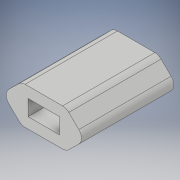
# Autodesk Inventor part: USB Plug Protector
Saved by Autodesk Inventor 2019 (Build 230136000, 136)
## iProperties
Created: 2021-08-13
Part Number: USB Plug Protector
Material: Generic
Document SubType Name: Modeling
Designer: Lix
Density: 1 g/cm^3
Appearance: Default
Author: Lix
Autodesk Inventor part; units mm, degrees
ref_plane "YZ Plane" through (0, 0, 0) normal (1, 0, 0) x (0, 1, 0)
ref_plane "XZ Plane" through (0, 0, 0) normal (0, 1, 0) x (-1, 0, 0)
ref_plane "XY Plane" through (0, 0, 0) normal (0, 0, 1) x (1, 0, 0)
sketch "Sketch1" plane through (0, 0, 0) normal (0, 0, 1) x (1, 0, 0)
  line L0 (-9.5418, 7) -> (9.5418, 7) construction
  arc A0 (-9.5418, 7) -> (-10.9418, 6.4283) centre (-9.5418, 5) ccw construction
  line L1 (-16.0429, 1.4283) -> (-10.9418, 6.4283) construction
  arc A1 (-16.0429, 1.4283) -> (-16.0429, -1.4283) centre (-14.6429, 0) ccw construction
  line L2 (-16.0429, -1.4283) -> (-10.9418, -6.4283) construction
  arc A2 (-10.9418, -6.4283) -> (-9.5418, -7) centre (-9.5418, -5) ccw construction
  line L3 (-9.5418, -7) -> (9.5418, -7) construction
  arc A3 (9.5418, -7) -> (10.9418, -6.4283) centre (9.5418, -5) ccw construction
  line L4 (16.0429, -1.4283) -> (10.9418, -6.4283) construction
  arc A4 (16.0429, -1.4283) -> (16.0429, 1.4283) centre (14.6429, 0) ccw construction
  line L5 (16.0429, 1.4283) -> (10.9418, 6.4283) construction
  arc A5 (10.9418, 6.4283) -> (9.5418, 7) centre (9.5418, 5) ccw construction
  line L6 (-6, -2) -> (6, -2) construction
  line L7 (-6, 2) -> (-6, -2) construction
  line L8 (6, 2) -> (-6, 2) construction
  line L9 (6, -2) -> (6, 2) construction
  line L10 (9.5418, 7.5) -> (-9.5418, 7.5)
  arc A6 (-9.5418, 7.5) -> (-11.2918, 6.7854) centre (-9.5418, 5) ccw
  line L11 (-11.2918, 6.7854) -> (-16.3929, 1.7854)
  arc A7 (-16.3929, 1.7854) -> (-16.3929, -1.7854) centre (-14.6429, 0) ccw
  line L12 (-16.3929, -1.7854) -> (-11.2918, -6.7854)
  arc A8 (-11.2918, -6.7854) -> (-9.5418, -7.5) centre (-9.5418, -5) ccw
  line L13 (-9.5418, -7.5) -> (9.5418, -7.5)
  arc A9 (9.5418, -7.5) -> (11.2918, -6.7854) centre (9.5418, -5) ccw
  line L14 (11.2918, -6.7854) -> (16.3929, -1.7854)
  arc A10 (16.3929, -1.7854) -> (16.3929, 1.7854) centre (14.6429, 0) ccw
  line L15 (16.3929, 1.7854) -> (11.2918, 6.7854)
  arc A11 (11.2918, 6.7854) -> (9.5418, 7.5) centre (9.5418, 5) ccw
  line L16 (-9.5418, 9.5) -> (9.5418, 9.5)
  arc A12 (12.6918, 8.2136) -> (9.5418, 9.5) centre (9.5418, 5) ccw
  line L17 (12.6918, 8.2136) -> (17.7929, 3.2136)
  arc A13 (17.7929, -3.2136) -> (17.7929, 3.2136) centre (14.6429, 0) ccw
  line L18 (17.7929, -3.2136) -> (12.6918, -8.2136)
  arc A14 (9.5418, -9.5) -> (12.6918, -8.2136) centre (9.5418, -5) ccw
  line L19 (9.5418, -9.5) -> (-9.5418, -9.5)
  arc A15 (-12.6918, -8.2136) -> (-9.5418, -9.5) centre (-9.5418, -5) ccw
  line L20 (-12.6918, -8.2136) -> (-17.7929, -3.2136)
  arc A16 (-17.7929, 3.2136) -> (-17.7929, -3.2136) centre (-14.6429, 0) ccw
  line L21 (-17.7929, 3.2136) -> (-12.6918, 8.2136)
  arc A17 (-9.5418, 9.5) -> (-12.6918, 8.2136) centre (-9.5418, 5) ccw
  line L22 (-6, 2) -> (6, -2) construction
  point P0 (0, 0)
  point P1 (17.5, -7)
  point P2 (0, 0)
  dimension "d0" = 0.5
  dimension "d1" = 2
  constraints: 46 end point, 36 point on circle, 18 centre point, 1 midpoint, 22 other
  measures "d0" distance between parallel lines of L0 L10
  measures "d1" distance between parallel lines of L10 L16
extrude "Extrusion1" add sketch "Sketch1" along normal blind 20
sketch "Sketch2" plane through (0, 0, 20) normal (0, 0, 1) x (1, 0, 0)
  line L0 (-9.5418, 7.5) -> (9.5418, 7.5) projected
  arc A0 (11.2918, 6.7854) -> (9.5418, 7.5) centre (9.5418, 5) ccw projected
  line L1 (11.2918, 6.7854) -> (16.3929, 1.7854) projected
  arc A1 (16.3929, -1.7854) -> (16.3929, 1.7854) centre (14.6429, 0) ccw projected
  line L2 (16.3929, -1.7854) -> (11.2918, -6.7854) projected
  arc A2 (9.5418, -7.5) -> (11.2918, -6.7854) centre (9.5418, -5) ccw projected
  line L3 (9.5418, -7.5) -> (-9.5418, -7.5) projected
  arc A3 (-11.2918, -6.7854) -> (-9.5418, -7.5) centre (-9.5418, -5) ccw projected
  line L4 (-11.2918, -6.7854) -> (-16.3929, -1.7854) projected
  arc A4 (-16.3929, 1.7854) -> (-16.3929, -1.7854) centre (-14.6429, 0) ccw projected
  line L5 (-16.3929, 1.7854) -> (-11.2918, 6.7854) projected
  arc A5 (-9.5418, 7.5) -> (-11.2918, 6.7854) centre (-9.5418, 5) ccw projected
  line L6 (-12.6918, 8.2136) -> (-17.7929, 3.2136) projected
  arc A6 (-17.7929, 3.2136) -> (-17.7929, -3.2136) centre (-14.6429, 0) ccw projected
  line L7 (-17.7929, -3.2136) -> (-12.6918, -8.2136) projected
  arc A7 (-12.6918, -8.2136) -> (-9.5418, -9.5) centre (-9.5418, -5) ccw projected
  line L8 (-9.5418, -9.5) -> (9.5418, -9.5) projected
  arc A8 (9.5418, -9.5) -> (12.6918, -8.2136) centre (9.5418, -5) ccw projected
  line L9 (12.6918, -8.2136) -> (17.7929, -3.2136) projected
  arc A9 (17.7929, -3.2136) -> (17.7929, 3.2136) centre (14.6429, 0) ccw projected
  line L10 (17.7929, 3.2136) -> (12.6918, 8.2136) projected
  arc A10 (12.6918, 8.2136) -> (9.5418, 9.5) centre (9.5418, 5) ccw projected
  line L11 (9.5418, 9.5) -> (-9.5418, 9.5) projected
  arc A11 (-9.5418, 9.5) -> (-12.6918, 8.2136) centre (-9.5418, 5) ccw projected
  line L12 (6, 2) -> (-6, 2) construction
  line L13 (6, -2) -> (6, 2) construction
  line L14 (-6, -2) -> (6, -2) construction
  line L15 (-6, 2) -> (-6, -2) construction
  line L16 (-6, 2) -> (6, 2) construction
  line L17 (6, 2) -> (6, -2) construction
  line L18 (6, -2) -> (-6, -2) construction
  line L19 (-6, -2) -> (-6, 2) construction
  line L20 (-8, 4) -> (8, 4)
  line L21 (8, 4) -> (8, -4)
  line L22 (8, -4) -> (-8, -4)
  line L23 (-8, -4) -> (-8, 4)
  line L24 (-8, 4) -> (8, -4) construction
  line L25 (8, 4) -> (-8, -4) construction
  point P0 (0, 0)
  dimension "d4" = 16
  dimension "d5" = 8
  constraints: 20 end point, 4 parallel, 2 horizontal, 2 midpoint, 2 perpendicular
  measures "d4" distance of L21.end L22.end
  measures "d5" distance of L20.end L21.end
extrude "Extrusion2" add sketch "Sketch2" along normal blind 2 contours L0 A0 L1 A1 L2 A2 L3 A3 L4 A4 L5 A5 | A11 L11 A10 L10 A9 L9 A8 L8 A7 L7 A6 L6
sketch "Sketch3" plane through (0, 0, 22) normal (0, 0, 1) x (1, 0, 0)
  line L0 (8, 4) -> (8, -4) projected
  line L1 (8, -4) -> (-8, -4) projected
  line L2 (-8, -4) -> (-8, 4) projected
  line L3 (-8, 4) -> (8, 4) projected
  line L4 (-12.6918, 8.2136) -> (-17.7929, 3.2136) projected
  arc A0 (-17.7929, 3.2136) -> (-17.7929, -3.2136) centre (-14.6429, 0) ccw projected
  line L5 (-17.7929, -3.2136) -> (-12.6918, -8.2136) projected
  arc A1 (-12.6918, -8.2136) -> (-9.5418, -9.5) centre (-9.5418, -5) ccw projected
  line L6 (-9.5418, -9.5) -> (9.5418, -9.5) projected
  arc A2 (9.5418, -9.5) -> (12.6918, -8.2136) centre (9.5418, -5) ccw projected
  line L7 (12.6918, -8.2136) -> (17.7929, -3.2136) projected
  arc A3 (17.7929, -3.2136) -> (17.7929, 3.2136) centre (14.6429, 0) ccw projected
  line L8 (17.7929, 3.2136) -> (12.6918, 8.2136) projected
  arc A4 (12.6918, 8.2136) -> (9.5418, 9.5) centre (9.5418, 5) ccw projected
  line L9 (9.5418, 9.5) -> (-9.5418, 9.5) projected
  arc A5 (-9.5418, 9.5) -> (-12.6918, 8.2136) centre (-9.5418, 5) ccw projected
  point P0 (0, 0)
extrude "Extrusion3" add sketch "Sketch3" along normal blind 25
body "Solid1"
